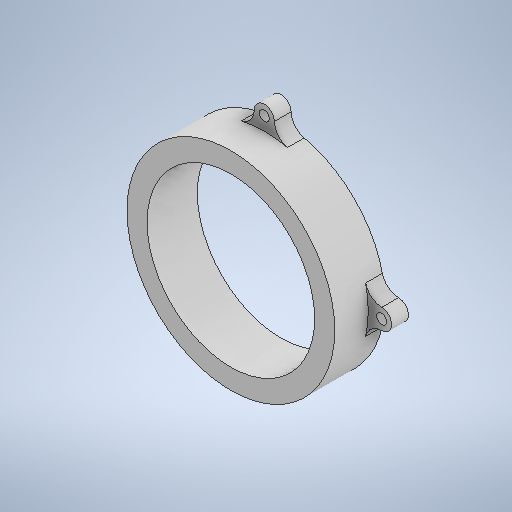
# Autodesk Inventor part: ModuleConnector
Saved by Autodesk Inventor 2025.1 (Build 291241020, 241B)
## iProperties
Created: 2024-09-22
Part Number: ModuleConnector
Material: 일반
Document SubType Name: Modeling
Designer: daare
Density: 1 g/cm^3
Appearance: 기본값
Author: daare
Autodesk Inventor part; units mm, degrees
ref_plane "YZ Plane" through (0, 0, 0) normal (1, 0, 0) x (0, 1, 0)
ref_plane "XZ Plane" through (0, 0, 0) normal (0, 1, 0) x (-1, 0, 0)
ref_plane "XY Plane" through (0, 0, 0) normal (0, 0, 1) x (1, 0, 0)
sketch "스케치1" plane through (0, 0, 0) normal (0, 0, 1) x (1, 0, 0)
  circle A0 centre (0, 0) radius 25
  arc A1 (-35.0375, 2.9998) -> (-35.0375, -2.9998) centre (-35, 0) ccw
  circle A2 centre (-35, 0) radius 1.5
  circle A3 centre (0, 0) radius 31
  arc A4 (-35.0375, 2.9998) -> (-30.225, 6.8884) centre (-35.1, 7.9994) ccw
  arc A5 (-30.225, -6.8884) -> (-35.0375, -2.9998) centre (-35.1, -7.9994) ccw
  circle A6 centre (0, -35) radius 1.5
  arc A7 (-2.9998, -35.0375) -> (2.9998, -35.0375) centre (0, -35) ccw
  arc A8 (-2.9998, -35.0375) -> (-6.8884, -30.225) centre (-7.9994, -35.1) ccw
  arc A9 (6.8884, -30.225) -> (2.9998, -35.0375) centre (7.9994, -35.1) ccw
  circle A10 centre (35, 0) radius 1.5
  arc A11 (35.0375, -2.9998) -> (35.0375, 2.9998) centre (35, 0) ccw
  arc A12 (35.0375, -2.9998) -> (30.225, -6.8884) centre (35.1, -7.9994) ccw
  arc A13 (30.225, 6.8884) -> (35.0375, 2.9998) centre (35.1, 7.9994) ccw
  circle A14 centre (0, 35) radius 1.5
  arc A15 (2.9998, 35.0375) -> (-2.9998, 35.0375) centre (0, 35) ccw
  arc A16 (2.9998, 35.0375) -> (6.8884, 30.225) centre (7.9994, 35.1) ccw
  arc A17 (-6.8884, 30.225) -> (-2.9998, 35.0375) centre (-7.9994, 35.1) ccw
  point P0 (30.225, 6.8884)
  point P1 (-6.8884, 30.225)
  dimension "d0" = 50
  dimension "d1" = 35
  dimension "d2" = 3
  dimension "d3" = 6
  dimension "d4" = 6
  dimension "d5" = 5
  dimension "d8" = 360
  constraints: 26 point on circle, 18 centre point, 5 coincident, 4 tangent, 1 equal radius, 1 horizontal alignment, 49 other
  measures "d0" diameter of A0
  measures "d1" distance of A1.centre point (0, 0)
  measures "d2" diameter of A2
  measures "d3" diameter of A1
  measures "d4" radial gap between concentric circles of A0 A3
  measures "d5" radius of A4
extrude "돌출1" add sketch "스케치1" along normal blind 5 contours A4 A3 A5 A1 | A17 A15 A16 A3 | A3 A9 A7 A8 | A13 A11 A12 A3
extrude "돌출2" add sketch "스케치1" along normal blind 15 contours A3
